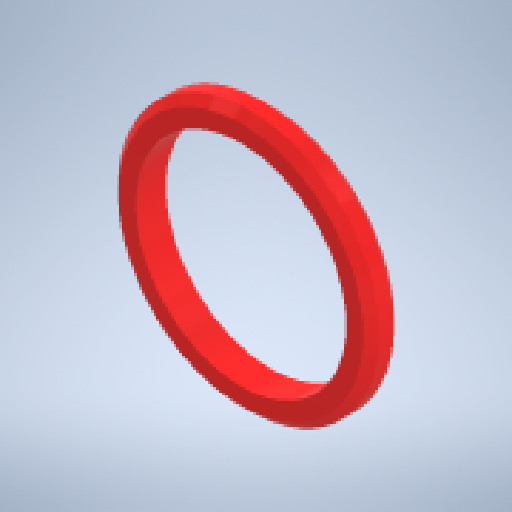
# Autodesk Inventor part: 出力ピンベアリングスペーサ2
Saved by Autodesk Inventor 2024 (Build 280153000, 153)
## iProperties
Created: 2023-06-01
Part Number: 出力ピンベアリングスペーサ2
Material: 一般
Document SubType Name: Modeling
Designer: yuta2
Density: 1 g/cm^3
Appearance: 淡い赤
Author: yuta2
Autodesk Inventor part; units mm, degrees
ref_plane "YZ Plane" through (0, 0, 0) normal (1, 0, 0) x (0, 1, 0)
ref_plane "XZ Plane" through (0, 0, 0) normal (0, 1, 0) x (-1, 0, 0)
ref_plane "XY Plane" through (0, 0, 0) normal (0, 0, 1) x (1, 0, 0)
sketch "スケッチ1" plane through (0, 0, 0) normal (0, 0, 1) x (1, 0, 0)
  circle A0 centre (0, 0) radius 5.25
  circle A1 centre (0, 0) radius 6.5
  dimension "d0" = 10.5
  dimension "d1" = 13
  constraints: 2 centre point, 2 coincident
  measures "d0" diameter of A0
  measures "d1" diameter of A1
extrude "押し出し1" add sketch "スケッチ1" along normal blind 1.5
chamfer "面取り1" distance 0.4 angle 45 2 edges at (-6.5, 0, 1.5) (-6.5, 0, 0)
